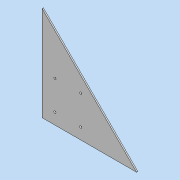
# Autodesk Inventor part: Display_CCM_Mount
Saved by Autodesk Inventor 2020 (Build 240168000, 168)
## iProperties
Created: 2021-07-12
Part Number: Display_CCM_Mount
Material: 一般
Document SubType Name: Sheet Metal
Designer: magnarecta
Density: 1 g/cm^3
Sheet Metal Rule: Default_mm
Appearance: 既定
Author: magnarecta
Autodesk Inventor part; units mm, degrees
ref_plane "YZ Plane" through (0, 0, 0) normal (1, 0, 0) x (0, 1, 0)
ref_plane "XZ Plane" through (0, 0, 0) normal (0, 1, 0) x (-1, 0, 0)
ref_plane "XY Plane" through (0, 0, 0) normal (0, 0, 1) x (1, 0, 0)
sketch "スケッチ1" plane through (0, 0, 0) normal (0, 0, 1) x (1, 0, 0)
  line L0 (0, 0) -> (220, 0)
  line L1 (220, 0) -> (220, 220)
  line L2 (220, 220) -> (0, 220)
  line L3 (0, 220) -> (0, 0)
  line L4 (0, 220) -> (220, 0)
  dimension "d0" = 220
  dimension "d1" = 220
  measures "d0" distance of L2.end L0.start
  measures "d1" distance of L0.start L0.end
extrude "プレート1" add sketch "スケッチ1" along normal blind 3 contours L3 L4 L0
sketch "スケッチ2" plane through (0, 0, 3) normal (0, 0, 1) x (1, 0, 0)
  line L0 (30, 26) -> (90, 26)
  line L1 (90, 26) -> (90, 94)
  line L2 (90, 94) -> (30, 94)
  line L3 (30, 94) -> (30, 26)
  line L4 (30, 26) -> (90, 94) construction
  line L5 (90, 26) -> (30, 94) construction
  line L6 (220, 0) -> (0, 0) projected
  line L7 (0, 0) -> (0, 220) projected
  point P0 (60, 60)
  dimension "d3" = 60
  dimension "d4" = 68
  dimension "d5" = 60
  dimension "d6" = 60
  constraints: 12 end point, 2 midpoint, 2 parallel, 1 horizontal, 1 perpendicular
  measures "d3" distance of L1.end L2.end
  measures "d4" distance of L0.end L1.end
  measures "d5" distance from line of point (60, 60) L6
  measures "d6" distance from line of point (60, 60) L7
hole "穴1" at (30, 26, 3) at (90, 26, 3) at (30, 94, 3) at (90, 94, 3) direction (0, 0, -1) diameter 5.2 depth 3 tip angle 118
equation "\"d12\" = Thickness"
equation "\"d2\" = Thickness"
equation "\"BendRadius\" = Thickness"
equation "\"BendReliefWidth\" = Thickness"
equation "\"BendReliefDepth\" = 0.5 * Thickness"
equation "\"CornerReliefSize\" = 4 * Thickness"
equation "\"MinimumRemnant\" = 2 * Thickness"
equation "\"TransitionRadius\" = BendRadius"
equation "\"JacobiRadiusSize\" = BendRadius"
equation "\"GapSize\" = Thickness"
equation "\"Thickness\" = 3"
